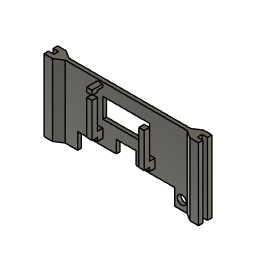
screen_holder v4 (Autodesk Fusion 360 design; units mm, degrees)
Autodesk Fusion 360 part; units mm, degrees
sketch "Sketch1" plane through (0, 0, 0) normal (0, 1, 0) x (1, 0, 0) in component "wire_organizer"
  line L0 (0, 0) -> (80, 0)
  line L1 (80, 0) -> (80, -40)
  line L2 (80, -40) -> (0, -40)
  line L3 (0, -40) -> (0, 0)
  line L4 (34.5, -16) -> (45.5, -16)
  line L5 (45.5, -16) -> (45.5, -9)
  line L6 (45.5, -9) -> (34.5, -9)
  line L7 (34.5, -9) -> (34.5, -16)
  circle A0 centre (71, -5) radius 2.5
  line L8 (27, -33) -> (53, -33)
  line L9 (53, -33) -> (53, -22)
  line L10 (53, -22) -> (27, -22)
  line L11 (27, -22) -> (27, -33)
  line L12 (40, -40) -> (40, -26) construction
  line L13 (67, 0) -> (13, 0)
  line L14 (13, 0) -> (13, -9)
  line L15 (13, -9) -> (67, -9)
  line L16 (67, -9) -> (67, 0)
  dimension "d1" = 80
  dimension "d2" = 40
  dimension "d3" = 11
  dimension "d4" = 7
  dimension "d5" = 5
  dimension "d6" = 26
  dimension "d7" = 11
  dimension "d9" = 5
  dimension "d15" = 54
  dimension "d16" = 9
  dimension "d17" = 6
  dimension "d42" = 4
  constraint horizontal L0
  constraint vertical L1
  constraint horizontal L2
  constraint vertical L3
  constraint coincident L0.start L3.end
  constraint horizontal L4
  constraint vertical L5
  constraint horizontal L6
  constraint vertical L7
  constraint horizontal L8
  constraint vertical L9
  constraint horizontal L10
  constraint vertical L11
  constraint midpoint L2 L12.start
  constraint perpendicular L10 L12
  constraint midpoint L8 L12
  constraint horizontal L13
  constraint vertical L14
  constraint horizontal L15
  constraint vertical L16
  constraint coincident L0 L13.start
  constraint midpoint L6 L15
  constraint midpoint L0 L13
  measures "d1" distance of L0.start L0.end
  measures "d2" distance of L0.start L2.end
  measures "d3" distance of L4.start L4.end
  measures "d4" distance of L4.start L6.end
  measures "d5" diameter of A0
  measures "d6" distance of L8.start L8.end
  measures "d7" distance of L8.start L10.end
  measures "d9" distance of L0 A0.centre
  measures "d15" distance of L13.start L13.end
  measures "d16" distance of L13.start L15.end
  measures "d17" distance of L4 L10
  measures "d42" distance of A0.centre L16
extrude "Extrude1" add sketch "Sketch1" along normal blind 2 contours L0 L1 L2 L3 L4 L5 L7 L14 L15 L16 makes body 1 in component "wire_organizer"
ref_plane "WorkPlane1" through (27, 1, 20) normal (-1, 0, 0) x (0, 0, 1) in component "wire_organizer"
sketch "Sketch3" plane through (27, 0, 0) normal (-1, 0, 0) x (0, -1, 0) in component "wire_organizer"
  line L0 (0, 14.7) -> (6, 14.7)
  line L1 (6, 14.7) -> (6, 17.7)
  line L2 (6, 17.7) -> (0, 17.7)
  line L3 (0, 17.7) -> (0, 14.7)
  line L4 (6, 17.7) -> (3, 17.7)
  line L5 (3, 17.7) -> (3, 34)
  line L6 (3, 34) -> (6, 34)
  line L7 (6, 34) -> (6, 17.7)
  line L8 (0, 0) -> (0, 40)
  line L9 (0, 14.7) -> (3, 14.7)
  line L10 (3, 14.7) -> (3, 12.7)
  line L11 (3, 12.7) -> (0, 12.7)
  line L12 (0, 12.7) -> (0, 14.7)
  line L13 (0, 22) -> (0, 33)
  line L14 (0, 39) -> (6, 39)
  line L15 (6, 39) -> (6, 37.5)
  line L16 (6, 37.5) -> (0, 37.5)
  line L17 (0, 37.5) -> (0, 39)
  line L18 (6, 37.5) -> (3, 37.5)
  line L19 (3, 37.5) -> (3, 36.5)
  line L20 (3, 36.5) -> (6, 36.5)
  line L21 (6, 36.5) -> (6, 37.5)
  point P0 (0, 22)
  dimension "d23" = 3
  dimension "d24" = 3
  dimension "d25" = 3
  dimension "d26" = 3
  dimension "d27" = 2
  dimension "d30" = 4.3
  dimension "d40" = 1.5
  dimension "d41" = 1
  constraint horizontal L0
  constraint vertical L1
  constraint horizontal L2
  constraint vertical L3
  constraint horizontal L4
  constraint vertical L5
  constraint horizontal L6
  constraint vertical L7
  constraint horizontal L9
  constraint vertical L10
  constraint horizontal L11
  constraint vertical L12
  constraint coincident L8 L0.start
  constraint coincident L0 L3.end
  constraint coincident L2.end L8
  constraint horizontal L14
  constraint vertical L15
  constraint horizontal L16
  constraint vertical L17
  constraint coincident L8 L14.start
  constraint horizontal L18
  constraint vertical L19
  constraint horizontal L20
  constraint vertical L21
  measures "d23" distance of L0.end L1.end
  measures "d24" distance of L5.end L6.end
  measures "d25" distance of L5 L8
  measures "d26" distance of L10.end L11.end
  measures "d27" distance of L9.end L10.end
  measures "d30" distance of L2.end P0
  measures "d40" distance of L14.end L15.end
  measures "d41" distance of L15.end L20.end
extrude "Extrude2" add sketch "Sketch3" along normal blind 3 separate body makes body 2 at (27, -5, 22.1333) makes body 3 at (26, -2, 39) in component "wire_organizer"
ref_plane "WorkPlane2" through (40, 1, 27.5) normal (-1, 0, 0) x (0, 0, 1) in component "wire_organizer"
mirror "Mirror1" about plane through (40, 1, 27.5) normal (-1, 0, 0) of bodies 2 makes body 4 in component "wire_organizer"
sketch "Sketch6" plane through (0, 0, 40) normal (0, 0, 1) x (-1, 0, 0) in component "wire_organizer"
  line L0 (-80, 0) -> (-80, -2)
  line L1 (0, -2) -> (-1.7287, -2)
  line L2 (-1.7287, -2) -> (-1.7287, -2.26)
  line L3 (-1.7287, -2.26) -> (0, -2.26)
  line L4 (0, -2.26) -> (0, -2)
  line L5 (-1.7287, -2.26) -> (3, -2.26)
  line L6 (3, -2.26) -> (3, -4.76)
  line L7 (3, -4.76) -> (-1.7287, -4.76)
  line L8 (-1.7287, -4.76) -> (-1.7287, -2.26)
  line L9 (0, 0) -> (0, -2)
  line L10 (0, -1) -> (3.7998, -1) construction
  line L11 (-1.7287, -4.76) -> (-6, -2)
  line L12 (0, -2) -> (-80, -2)
  line L13 (-1.7287, 2.76) -> (-6, 0)
  line L14 (-1.7287, 2.76) -> (-1.7287, 0.26)
  line L15 (3, 2.76) -> (-1.7287, 2.76)
  line L16 (3, 0.26) -> (3, 2.76)
  line L17 (-1.7287, 0.26) -> (3, 0.26)
  line L18 (0, 0) -> (-1.7287, 0)
  line L19 (-1.7287, 0) -> (-1.7287, 0.26)
  line L20 (0, 0.26) -> (0, 0)
  line L21 (-80, 0) -> (0, 0)
  line L22 (-40, -2) -> (-40, -11) construction
  line L23 (-40, -2) -> (-40, -11) construction
  line L24 (-78.2713, -4.76) -> (-74, -2)
  line L25 (-80, -2.26) -> (-80, -2)
  line L26 (0, 0) -> (-80, 0)
  line L27 (-78.2713, -4.76) -> (-78.2713, -2.26)
  line L28 (-83, 0.26) -> (-83, 2.76)
  line L29 (-78.2713, -2.26) -> (-83, -2.26)
  line L30 (-78.2713, 0.26) -> (-83, 0.26)
  line L31 (-78.2713, -2) -> (-78.2713, -2.26)
  line L32 (-80, 0.26) -> (-80, 0)
  line L33 (-83, 2.76) -> (-78.2713, 2.76)
  line L34 (-78.2713, 0) -> (-78.2713, 0.26)
  line L35 (-78.2713, 2.76) -> (-74, 0)
  line L36 (-80, 0) -> (-78.2713, 0)
  line L37 (-80, -2) -> (0, -2)
  line L38 (-78.2713, 2.76) -> (-78.2713, 0.26)
  line L39 (-80, -2) -> (-78.2713, -2)
  line L40 (-78.2713, -2.26) -> (-80, -2.26)
  line L41 (-80, 0) -> (-80, -2)
  line L42 (-83, -4.76) -> (-78.2713, -4.76)
  line L43 (-83, -2.26) -> (-83, -4.76)
  line L44 (-80, -1) -> (-83.7998, -1) construction
  point P0 (-80, 0)
  dimension "d36" = 1.26
  dimension "d37" = 2.5
  constraint horizontal L1
  constraint vertical L2
  constraint horizontal L3
  constraint vertical L4
  constraint horizontal L5
  constraint vertical L6
  constraint horizontal L7
  constraint vertical L8
  constraint midpoint L9 L10.start
  constraint perpendicular L9 L10
  constraint coincident L11.end L12
  constraint symmetric L1.start L10 L9.start
  constraint symmetric L1.end L10 L18.end
  constraint symmetric L2.end L10 L14.end
  constraint symmetric L3.end L10 L20.start
  constraint symmetric L5.end L10 L16.start
  constraint symmetric L6.end L10 L15.start
  constraint symmetric L7.end L10 L13.start
  constraint symmetric L10 L11.end L13.end
  constraint midpoint L12 L22.start
  constraint perpendicular L12 L22
  constraint symmetric L9.start L22 L0.start
  constraint symmetric L1.start L22 L0.end
  constraint symmetric L1.end L22 L31.start
  constraint symmetric L2.end L22 L27.end
  constraint symmetric L3.end L22 L25.start
  constraint symmetric L5.end L22 L29.end
  constraint symmetric L6.end L22 L42.start
  constraint symmetric L7.end L22 L24.start
  constraint symmetric L9.start L22 P0
  constraint symmetric L10.start L22 L44.start
  constraint symmetric L10.end L22 L44.end
  constraint symmetric L11.end L22 L24.end
  constraint symmetric L0.end L22 L1.start
  constraint symmetric L13.start L22 L33.end
  constraint symmetric L13.end L22 L35.end
  constraint symmetric L14.end L22 L30.start
  constraint symmetric L15.start L22 L28.end
  constraint symmetric L16.start L22 L28.start
  constraint symmetric L18.end L22 L34.start
  constraint symmetric L20.start L22 L32.start
  constraint symmetric P0 L22 L9.start
  constraint symmetric L23.start L22 L22.start
  constraint symmetric L23.end L22 L22.end
  measures "d36" distance of L5 L10
  measures "d37" distance of L2.end L7.end
extrude "Extrude4" add sketch "Sketch6" against normal up to surface (40 mm away) contours L21 L26 L30 L32 L34 L36 | L12 L25 L29 L31 L37 L39 L40 | L21 L26 L34 L35 L38 | L28 L30 L33 L38 | L12 L24 L27 L31 L37 | L27 L29 L40 L42 L43 | L13 L14 L19 L21 L26 | L2 L8 L11 L12 L37 | L14 L15 L16 L17 | L17 L18 L19 L20 L21 L26 | L3 L5 L6 L7 L8 | L1 L2 L3 L4 L5 L12 L37 bodies 1 in component "wire_organizer"
component "wire_organizer" placed x (1, 0, 0) y (0, 1, 0) z (0, 0, 1) at (0, 0, 0)
equation "d24 = d23"
equation "d26 = d23"
equation "d36 = ( 2.52 / 2 ) * 1 mm"
